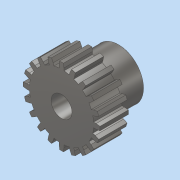
# Autodesk Inventor part: PinionGear20T
Saved by Autodesk Inventor 2017 (Build 210142000, 142)
## iProperties
Created: 2018-04-08
Part Number: PinionGear20T
Material: Stainless Steel
Document SubType Name: Modeling
Designer: Derek Wider
Density: 8 g/cm^3
Appearance: Semi-Polished
Author: Derek Wider
Autodesk Inventor part; units mm, degrees
ref_plane "YZ Plane" through (0, 0, 0) normal (1, 0, 0) x (0, 1, 0)
ref_plane "XZ Plane" through (0, 0, 0) normal (0, 1, 0) x (-1, 0, 0)
ref_plane "XY Plane" through (0, 0, 0) normal (0, 0, 1) x (1, 0, 0)
sketch "Sketch1" plane through (0, 0, 0) normal (0, 0, 1) x (1, 0, 0)
  circle A0 centre (0, 0) radius 3.81
  dimension "d0" = 7.62
  constraints: 1 centre point, 1 coincident
  measures "d0" diameter of A0
extrude "Extrusion1" add sketch "Sketch1" along normal blind 4.318
sketch "Sketch2" plane through (0, 0, 4.318) normal (0, 0, 1) x (1, 0, 0)
  circle A0 centre (0, 0) radius 4.8768
  dimension "d3" = 9.7536
  constraints: 1 centre point, 1 coincident
  measures "d3" diameter of A0
extrude "Extrusion2" add sketch "Sketch2" along normal blind 4.318
sketch "Sketch3" plane through (0, 0, 8.636) normal (0, 0, 1) x (1, 0, 0)
  line L0 (-0.3683, 4.8629) -> (-0.3683, 5.2439)
  line L1 (-0.3683, 5.2439) -> (-0.2921, 5.8281)
  line L2 (-0.2921, 5.8281) -> (0.2921, 5.8281)
  line L3 (0.2921, 5.8281) -> (0.3683, 5.2439)
  line L4 (0.3683, 5.2439) -> (0.3683, 4.8629)
  line L5 (0.3683, 4.8629) -> (-0.3683, 4.8629)
  circle A0 centre (0, 0) radius 4.8768 projected
  point P0 (0, 5.8281)
  point P1 (0, 4.8629)
  dimension "d6" = 0.7366
  dimension "d7" = 0.5842
  dimension "d8" = 0.381
  dimension "d9" = 0.5842
  constraints: 12 end point, 2 midpoint, 2 perpendicular, 2 vertical alignment, 1 horizontal alignment, 1 parallel, 1 vertical, 2 other
  measures "d6" distance of L4.end L0.start
  measures "d7" distance of L1.end L2.end
  measures "d8" distance of L0.start L0.end
  measures "d9" vertical distance of L0.end L1.end
extrude "Extrusion3" add sketch "Sketch3" against normal up to surface (4.318 mm away) contours A0 L5 | L0 L1 L2 L3 L4 A0 picked at (-0.041, 4.867)
pattern_circular "Circular Pattern1" count 20 over 360 about axis through (0, 0, 4.318) along (0, 0, 1) of "Extrusion3"
sketch "Sketch4" plane through (0, 0, 8.636) normal (0, 0, 1) x (1, 0, 0)
  circle A0 centre (0, 0) radius 1.5875
  dimension "d15" = 3.175
  constraints: 1 centre point, 1 coincident
  measures "d15" diameter of A0
extrude "Extrusion4" cut sketch "Sketch4" against normal through all
sketch "Sketch5" plane through (0, 0, 0) normal (0, 0, -1) x (-1, 0, 0)
  line L0 (-2.2445, 2.8767) -> (2.1991, 2.8767) construction
  line L1 (2.1991, 2.8767) -> (2.1991, 1.9463) construction
  line L2 (2.1991, 1.9463) -> (-2.2445, 1.9463) construction
  line L3 (-2.2445, 1.9463) -> (-2.2445, 2.8767) construction
  line L4 (-1.6307, 1.9665) -> (-2.1796, 1.9665)
  line L5 (-2.1796, 1.9665) -> (-2.1796, 2.0927)
  spline S0 degree 2 poles (-2.1796, 2.0927) (-2.1204, 2.1482) (-2.0151, 2.2514) (-1.9646, 2.3069) knots 0 0 0 1 2 2 2
  spline S1 degree 2 poles (-1.9646, 2.3069) (-1.8629, 2.4187) (-1.7886, 2.5528) (-1.7886, 2.6242) knots 0 0 0 1 2 2 2
  spline S2 degree 2 poles (-1.7886, 2.6242) (-1.7886, 2.6618) (-1.8117, 2.718) (-1.8326, 2.736) knots 0 0 0 1 2 2 2
  spline S3 degree 2 poles (-1.8326, 2.736) (-1.8536, 2.7541) (-1.9084, 2.7721) (-1.9415, 2.7721) knots 0 0 0 1 2 2 2
  spline S4 degree 2 poles (-1.9415, 2.7721) (-1.9733, 2.7721) (-2.0382, 2.7562) (-2.0678, 2.744) knots 0 0 0 1 2 2 2
  spline S5 degree 2 poles (-2.0678, 2.744) (-2.093, 2.7339) (-2.1399, 2.705) (-2.1543, 2.6949) knots 0 0 0 1 2 2 2
  line L6 (-2.1543, 2.6949) -> (-2.1608, 2.6949)
  line L7 (-2.1608, 2.6949) -> (-2.1608, 2.8219)
  spline S6 degree 2 poles (-2.1608, 2.8219) (-2.124, 2.8399) (-1.992, 2.8752) (-1.9329, 2.8752) knots 0 0 0 1 2 2 2
  spline S7 degree 2 poles (-1.9329, 2.8752) (-1.8081, 2.8752) (-1.6675, 2.7433) (-1.6675, 2.6307) knots 0 0 0 1 2 2 2
  spline S8 degree 2 poles (-1.6675, 2.6307) (-1.6675, 2.5781) (-1.692, 2.4901) (-1.7136, 2.4526) knots 0 0 0 1 2 2 2
  spline S9 degree 2 poles (-1.7136, 2.4526) (-1.7353, 2.4136) (-1.798, 2.3372) (-1.8326, 2.3004) knots 0 0 0 1 2 2 2
  spline S10 degree 2 poles (-1.8326, 2.3004) (-1.8889, 2.2391) (-2.0267, 2.1078) (-2.0678, 2.0696) knots 0 0 0 1 2 2 2
  line L8 (-2.0678, 2.0696) -> (-1.6307, 2.0696)
  line L9 (-1.6307, 2.0696) -> (-1.6307, 1.9665)
  spline S11 degree 2 poles (-0.9578, 2.4115) (-0.9578, 2.172) (-1.097, 1.9477) (-1.2419, 1.9477) knots 0 0 0 1 2 2 2
  spline S12 degree 2 poles (-1.2419, 1.9477) (-1.3891, 1.9477) (-1.5268, 2.1764) (-1.5268, 2.4108) knots 0 0 0 1 2 2 2
  spline S13 degree 2 poles (-1.5268, 2.4108) (-1.5268, 2.6517) (-1.3876, 2.8745) (-1.2419, 2.8745) knots 0 0 0 1 2 2 2
  spline S14 degree 2 poles (-1.2419, 2.8745) (-1.0955, 2.8745) (-0.9578, 2.6437) (-0.9578, 2.4115) knots 0 0 0 1 2 2 2
  spline S15 degree 2 poles (-1.1107, 2.1403) (-1.0934, 2.1843) (-1.0789, 2.3199) (-1.0789, 2.4115) knots 0 0 0 1 2 2 2
  spline S16 degree 2 poles (-1.0789, 2.4115) (-1.0789, 2.5031) (-1.0934, 2.638) (-1.1114, 2.6834) knots 0 0 0 1 2 2 2
  spline S17 degree 2 poles (-1.1114, 2.6834) (-1.1294, 2.7288) (-1.1922, 2.7757) (-1.2419, 2.7757) knots 0 0 0 1 2 2 2
  spline S18 degree 2 poles (-1.2419, 2.7757) (-1.2917, 2.7757) (-1.3559, 2.7288) (-1.3746, 2.6819) knots 0 0 0 1 2 2 2
  spline S19 degree 2 poles (-1.3746, 2.6819) (-1.3927, 2.6365) (-1.4057, 2.498) (-1.4057, 2.4108) knots 0 0 0 1 2 2 2
  spline S20 degree 2 poles (-1.4057, 2.4108) (-1.4057, 2.317) (-1.3941, 2.1915) (-1.3754, 2.1425) knots 0 0 0 1 2 2 2
  spline S21 degree 2 poles (-1.3754, 2.1425) (-1.3581, 2.0963) (-1.2939, 2.0465) (-1.2419, 2.0465) knots 0 0 0 1 2 2 2
  spline S22 degree 2 poles (-1.2419, 2.0465) (-1.1929, 2.0465) (-1.1287, 2.0934) (-1.1107, 2.1403) knots 0 0 0 1 2 2 2
  line L10 (-0.6109, 1.9665) -> (-0.6109, 2.7512)
  line L11 (-0.6109, 2.7512) -> (-0.9094, 2.7512)
  line L12 (-0.9094, 2.7512) -> (-0.9094, 2.8565)
  line L13 (-0.9094, 2.8565) -> (-0.194, 2.8565)
  line L14 (-0.194, 2.8565) -> (-0.194, 2.7512)
  line L15 (-0.194, 2.7512) -> (-0.4926, 2.7512)
  line L16 (-0.4926, 2.7512) -> (-0.4926, 1.9665)
  line L17 (-0.4926, 1.9665) -> (-0.6109, 1.9665)
  line L18 (0.8259, 2.2723) -> (0.7198, 2.2723)
  line L19 (0.7198, 2.2723) -> (0.7198, 1.9665)
  line L20 (0.7198, 1.9665) -> (0.6052, 1.9665)
  line L21 (0.6052, 1.9665) -> (0.6052, 2.2723)
  line L22 (0.6052, 2.2723) -> (0.2121, 2.2723)
  line L23 (0.2121, 2.2723) -> (0.2121, 2.3978)
  line L24 (0.2121, 2.3978) -> (0.6102, 2.8565)
  line L25 (0.6102, 2.8565) -> (0.7198, 2.8565)
  line L26 (0.7198, 2.8565) -> (0.7198, 2.3682)
  line L27 (0.7198, 2.3682) -> (0.8259, 2.3682)
  line L28 (0.8259, 2.3682) -> (0.8259, 2.2723)
  line L29 (0.6052, 2.3682) -> (0.6052, 2.7158)
  line L30 (0.6052, 2.7158) -> (0.3059, 2.3682)
  line L31 (0.3059, 2.3682) -> (0.6052, 2.3682)
  spline S23 degree 2 poles (1.1901, 1.9463) (1.1237, 1.9463) (1.0148, 1.9859) (0.9766, 2.0227) knots 0 0 0 1 2 2 2
  spline S24 degree 2 poles (0.9766, 2.0227) (0.9391, 2.0588) (0.9002, 2.1569) (0.9002, 2.2124) knots 0 0 0 1 2 2 2
  spline S25 degree 2 poles (0.9002, 2.2124) (0.9002, 2.2845) (0.9773, 2.4057) (1.0509, 2.4418) knots 0 0 0 1 2 2 2
  line L32 (1.0509, 2.4418) -> (1.0509, 2.4454)
  spline S26 degree 2 poles (1.0509, 2.4454) (0.9853, 2.4836) (0.9218, 2.5745) (0.9218, 2.6423) knots 0 0 0 1 2 2 2
  spline S27 degree 2 poles (0.9218, 2.6423) (0.9218, 2.7425) (1.0733, 2.8767) (1.1901, 2.8767) knots 0 0 0 1 2 2 2
  spline S28 degree 2 poles (1.1901, 2.8767) (1.3113, 2.8767) (1.4577, 2.7497) (1.4577, 2.6502) knots 0 0 0 1 2 2 2
  spline S29 degree 2 poles (1.4577, 2.6502) (1.4577, 2.5903) (1.3877, 2.4735) (1.3221, 2.4403) knots 0 0 0 1 2 2 2
  line L33 (1.3221, 2.4403) -> (1.3221, 2.4367)
  spline S30 degree 2 poles (1.3221, 2.4367) (1.4, 2.4007) (1.48, 2.2968) (1.48, 2.2146) knots 0 0 0 1 2 2 2
  spline S31 degree 2 poles (1.48, 2.2146) (1.48, 2.1006) (1.3142, 1.9463) (1.1901, 1.9463) knots 0 0 0 1 2 2 2
  spline S32 degree 2 poles (1.3574, 2.203) (1.3574, 2.2579) (1.3142, 2.3228) (1.2528, 2.3559) knots 0 0 0 1 2 2 2
  spline S33 degree 2 poles (1.2528, 2.3559) (1.2327, 2.3675) (1.1649, 2.3942) (1.1223, 2.4115) knots 0 0 0 1 2 2 2
  spline S34 degree 2 poles (1.1223, 2.4115) (1.0733, 2.379) (1.0206, 2.2824) (1.0206, 2.2211) knots 0 0 0 1 2 2 2
  spline S35 degree 2 poles (1.0206, 2.2211) (1.0206, 2.1403) (1.118, 2.035) (1.1915, 2.035) knots 0 0 0 1 2 2 2
  spline S36 degree 2 poles (1.1915, 2.035) (1.2665, 2.035) (1.3574, 2.1251) (1.3574, 2.203) knots 0 0 0 1 2 2 2
  spline S37 degree 2 poles (1.3408, 2.6488) (1.3408, 2.7086) (1.2608, 2.7887) (1.1894, 2.7887) knots 0 0 0 1 2 2 2
  spline S38 degree 2 poles (1.1894, 2.7887) (1.1245, 2.7887) (1.0415, 2.7173) (1.0415, 2.656) knots 0 0 0 1 2 2 2
  spline S39 degree 2 poles (1.0415, 2.656) (1.0415, 2.612) (1.0841, 2.5507) (1.1266, 2.5262) knots 0 0 0 1 2 2 2
  spline S40 degree 2 poles (1.1266, 2.5262) (1.1447, 2.5161) (1.2211, 2.4807) (1.2521, 2.4706) knots 0 0 0 1 2 2 2
  spline S41 degree 2 poles (1.2521, 2.4706) (1.3041, 2.5103) (1.3408, 2.5947) (1.3408, 2.6488) knots 0 0 0 1 2 2 2
  spline S42 degree 2 poles (2.1768, 2.5882) (2.1768, 2.5305) (2.1356, 2.4266) (2.0989, 2.3906) knots 0 0 0 1 2 2 2
  spline S43 degree 2 poles (2.0989, 2.3906) (2.0527, 2.3451) (1.9279, 2.2982) (1.8327, 2.2982) knots 0 0 0 1 2 2 2
  line L34 (1.8327, 2.2982) -> (1.7325, 2.2982)
  line L35 (1.7325, 2.2982) -> (1.7325, 1.9665)
  line L36 (1.7325, 1.9665) -> (1.6142, 1.9665)
  line L37 (1.6142, 1.9665) -> (1.6142, 2.8565)
  line L38 (1.6142, 2.8565) -> (1.8378, 2.8565)
  spline S44 degree 2 poles (1.8378, 2.8565) (1.9171, 2.8565) (2.0282, 2.8305) (2.0707, 2.801) knots 0 0 0 1 2 2 2
  spline S45 degree 2 poles (2.0707, 2.801) (2.1205, 2.7671) (2.1768, 2.6625) (2.1768, 2.5882) knots 0 0 0 1 2 2 2
  spline S46 degree 2 poles (2.0534, 2.5846) (2.0534, 2.6307) (2.0217, 2.6985) (1.9892, 2.7202) knots 0 0 0 1 2 2 2
  spline S47 degree 2 poles (1.9892, 2.7202) (1.9611, 2.7389) (1.8861, 2.7541) (1.8306, 2.7541) knots 0 0 0 1 2 2 2
  line L39 (1.8306, 2.7541) -> (1.7325, 2.7541)
  line L40 (1.7325, 2.7541) -> (1.7325, 2.3992)
  line L41 (1.7325, 2.3992) -> (1.8133, 2.3992)
  spline S48 degree 2 poles (1.8133, 2.3992) (1.8854, 2.3992) (1.9741, 2.4223) (2.0029, 2.4526) knots 0 0 0 1 2 2 2
  spline S49 degree 2 poles (2.0029, 2.4526) (2.0296, 2.4793) (2.0534, 2.542) (2.0534, 2.5846) knots 0 0 0 1 2 2 2
  point P0 (0, 0)
  constraints: 2 other
emboss "Emboss1" sketch "Sketch5" operation cut depth 0.254 direction (0, 0, 1)
body "Solid1"
